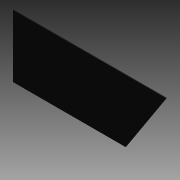
# Autodesk Inventor part: side shell model
Saved by Autodesk Inventor 2012 (Build 160160000, 160)
## iProperties
Created: 2011-12-30
Part Number: side shell model
Material: Default
Document SubType Name: Modeling
Designer: Antonella
Density: 1 g/cm^3
Author: Antonella
Autodesk Inventor part; units mm, degrees
ref_plane "YZ Plane" through (0, 0, 0) normal (1, 0, 0) x (0, 1, 0)
ref_plane "XZ Plane" through (0, 0, 0) normal (0, 1, 0) x (-1, 0, 0)
ref_plane "XY Plane" through (0, 0, 0) normal (0, 0, 1) x (1, 0, 0)
sketch "Sketch1" plane through (0, 0, 0) normal (0, 0, 1) x (1, 0, 0)
  line L0 (-353.06, 0) -> (518.16, 0) projected
  line L1 (0, -177.8) -> (0, 177.8) projected
  line L2 (-228.6, 127) -> (393.7, 127)
  line L3 (393.7, 127) -> (228.6, -127)
  line L4 (228.6, -127) -> (-228.6, -127)
  line L5 (-228.6, -127) -> (-228.6, 127)
  point P0 (0, 0)
  point P1 (-228.6, 0)
  point P2 (0, -127)
  dimension "d0" = 254
  dimension "d1" = 457.2
  dimension "d2" = 622.3
  constraints: 8 end point, 2 midpoint, 2 perpendicular, 1 horizontal alignment, 1 parallel, 1 vertical alignment
  measures "d0" distance of L4.end L2.start
  measures "d1" distance of L3.end L4.end
  measures "d2" distance of L2.start L2.end
extrude "Extrusion1" add sketch "Sketch1" along normal blind 3.175
body "Solid1"
